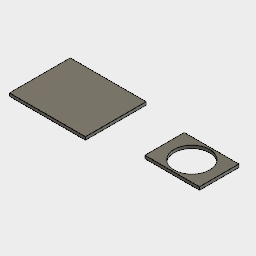
LED Strip Boxes V1 v8 (Autodesk Fusion 360 design; units mm, degrees)
Autodesk Fusion 360 part; units mm, degrees
note: some values were not read from the file. Set by a fixed rule: which face or edge a step refers to.
sketch "Sketch1" plane through (0, 0, 0) normal (0, 1, 0) x (1, 0, 0)
  line L0 (0, 0) -> (48, 0)
  line L1 (48, 0) -> (48, -40)
  line L2 (48, -40) -> (0, -40)
  line L3 (0, -40) -> (0, 0)
  dimension "d1" = 40
  dimension "d2" = 48
  measures "d1" distance of L0.start L2.end
  measures "d2" distance of L0.start L0.end
extrude "Extrude2" add sketch "Sketch1" along normal blind 33 makes body 1
shell "Shell2" thickness 3 removed faces 1 at (16, 33, 26.6667) on bodies 1
sketch "Sketch2" plane through (0, 0, 0) normal (0, 1, 0) x (1, 0, 0)
  line L0 (60, 0) -> (92, 0)
  line L1 (92, 0) -> (92, -24)
  line L2 (92, -24) -> (60, -24)
  line L3 (60, -24) -> (60, 0)
  dimension "d9" = 32
  dimension "d10" = 24
  measures "d9" distance of L0.start L0.end
  measures "d10" distance of L0.start L2.end
extrude "Extrude3" add sketch "Sketch2" along normal blind 10 separate body makes body 2
shell "Shell3" thickness 2 outward yes removed faces 1 at (70.6667, 10, 8) on bodies 2
move_face "OffsetFaces1" offset -1 1 faces at (32, 11, 40) on bodies 1
move_face "OffsetFaces2" offset -1 3 faces at (16, 11, 0) (0, 11, 26) (48, 11, 13) on bodies 1
move_body "Move1" bodies 2 to x (1, 0, 0) y (0, 1, 0) z (0, 0, 1) at (20, 0, 0)
extrude "Extrude4" cut 1 faces at (112, 3.3333, 8) along direction (1, 0, 0) blind 0.25 on bodies 2 bodies 2
extrude "Extrude5" cut 1 faces at (80, 3.3333, 16) along direction (-1, 0, 0) blind 0.25 on bodies 2 bodies 2
extrude "Extrude6" cut 1 faces at (101.4167, 6.6667, 0) along direction (0, 0, -1) blind 0.05 on bodies 2 bodies 2
extrude "Extrude7" add 1 faces at (101.4167, 3.3333, 24) along direction (0, 0, -1) blind 0.05 on bodies 2 bodies 2
extrude "Extrude8" cut 1 faces at (101.4167, 6.6667, -0.05) along direction (0, 0, -1) blind 0.05 on bodies 2 bodies 2
extrude "Extrude9" cut 1 faces at (101.4167, 3.3333, 23.95) along direction (0, 0, 1) blind 0.05 on bodies 2 bodies 2
extrude "Extrude10" add 1 faces at (1, 11, 26.3333) along direction (-1, 0, 0) blind 2 on bodies 1 bodies 1
extrude "Extrude11" add 1 faces at (47, 11, 13.6667) along direction (1, 0, 0) blind 2 on bodies 1 bodies 1
extrude "Extrude12" cut 1 faces at (3, 23, 14.3333) along direction (-1, 0, 0) blind 2 on bodies 1 bodies 1
extrude "Extrude13" cut 1 faces at (45, 23, 25.6667) along direction (1, 0, 0) blind 2 on bodies 1 bodies 1
extrude "Extrude14" cut 1 faces at (47, 23, 25.6667) along direction (1, 0, 0) blind 0.1 on bodies 1 bodies 1
extrude "Extrude15" cut 1 faces at (1, 23, 14.3333) along direction (-1, 0, 0) blind 0.1 on bodies 1 bodies 1
extrude "Extrude16" add 1 faces at (32.3333, 11, 39) along direction (0, 0, 1) blind 1 on bodies 1 bodies 1
extrude "Extrude17" cut 1 faces at (31.7, 13, 3) along direction (0, 0, -1) blind 1 on bodies 1 bodies 1
extrude "Extrude18" cut 1 faces at (16.3, 13, 37) along direction (0, 0, 1) blind 1 on bodies 1 bodies 1
extrude "Extrude19" add 1 faces at (32.3333, 11, 1) along direction (0, 0, -1) blind 1 on bodies 1 bodies 1
extrude "Extrude20" cut 1 faces at (16.3, 13, 38) along direction (0, 0, 1) blind 0.4 on bodies 1 bodies 1
extrude "Extrude21" cut 1 faces at (31.7, 13, 2) along direction (0, 0, -1) blind 0.4 on bodies 1 bodies 1
extrude "Extrude22" cut 1 faces at (31.7, 13, 1.6) along direction (0, 0, -1) blind 0.1 on bodies 1 bodies 1
extrude "Extrude23" cut 1 faces at (16.3, 13, 38.4) along direction (0, 0, 1) blind 0.1 on bodies 1 bodies 1
move_face "OffsetFaces3" offset 3 1 faces at (101.4167, 10, 25.3333) on bodies 2
extrude "Extrude24" cut 1 faces at (101.4167, 8.6667, -0.1) along direction (0, 0, -1) blind 0.1 on bodies 2 bodies 2
extrude "Extrude25" cut 1 faces at (79.75, 4.3333, 7.8667) along direction (-1, 0, 0) blind 0.1 on bodies 2 bodies 2
extrude "Extrude26" cut 1 faces at (90.5167, 8.6667, 24) along direction (0, 0, 1) blind 0.1 on bodies 2 bodies 2
extrude "Extrude27" cut 1 faces at (112.25, 4.3333, 16) along direction (1, 0, 0) blind 0.1 on bodies 2 bodies 2
extrude "Extrude28" cut 1 faces at (112.35, 4.3333, 16) along direction (1, 0, 0) blind 0.15 on bodies 2 bodies 2
extrude "Extrude29" cut 1 faces at (79.65, 4.3333, 7.9) along direction (-1, 0, 0) blind 0.15 on bodies 2 bodies 2
extrude "Extrude30" cut 1 faces at (90.5, 4.3333, 24.1) along direction (0, 0, 1) blind 0.25 on bodies 2 bodies 2
extrude "Extrude31" cut 1 faces at (101.5, 8.6667, -0.2) along direction (0, 0, -1) blind 0.25 on bodies 2 bodies 2
sketch "Sketch3" plane through (0, 0, 0) normal (0, 1, 0) x (1, 0, 0)
move_face "MoveFace1" by (0, 0, 20) 1 faces at (90.5, 0, 7.8167) on bodies 2
sketch "Sketch4" plane through (0, 0, 0) normal (0, 1, 0) x (-1, 0, 0)
  line L0 (-79.5, -0.45) -> (-79.5, 24.35)
  line L1 (-79.5, 24.35) -> (-112.5, 24.35)
  line L2 (-112.5, 24.35) -> (-112.5, -0.45)
  line L3 (-112.5, -0.45) -> (-79.5, -0.45)
  line L4 (-78, -2) -> (-114, -2)
  line L5 (-114, -2) -> (-114, 26)
  line L6 (-114, 26) -> (-78, 26)
  line L7 (-78, 26) -> (-78, -2)
  line L8 (-80, 35) -> (-116, 35)
  line L9 (-116, 35) -> (-116, 61)
  line L10 (-116, 61) -> (-80, 61)
  line L11 (-80, 61) -> (-80, 35)
  line L12 (0, 50) -> (-50, 50)
  line L13 (-50, 50) -> (-50, 90)
  line L14 (-50, 90) -> (0, 90)
  line L15 (0, 90) -> (0, 50)
  line L16 (-98, 35) -> (-98, 61)
  circle A0 centre (-98, 48) radius 11.65
  point P0 (-78, -2)
  point P1 (-114, 26)
  dimension "d80" = 36
  dimension "d81" = 26
  dimension "d82" = 50
  dimension "d83" = 40
  dimension "d84" = 23.3
  measures "d80" distance of L8.start L8.end
  measures "d81" distance of L8.start L10.end
  measures "d82" distance of L12.start L12.end
  measures "d83" distance of L12.start L14.end
  measures "d84" diameter of A0
extrude "Extrude32" add sketch "Sketch4" along normal blind 2 separate body contours L8 L10 L11 L16 A0 | L8 L9 L10 L16 A0 makes body 3
extrude "Extrude33" add sketch "Sketch4" along normal blind 2 separate body contours L12 L13 L14 L15 makes body 4
move_body "Move2" bodies 3 to x (1, 0, 0) y (0, 1, 0) z (0, 0, 1) at (0, 0, 20)
shell "Shell1" [suppressed]
extrude "Extrude1" [suppressed]
hidden bodies 1 2
